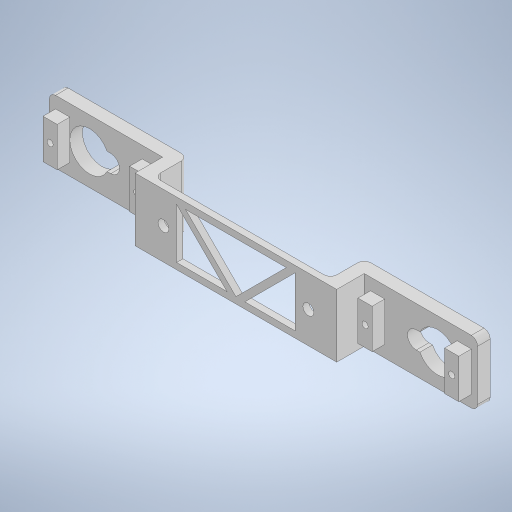
# Autodesk Inventor part: axis2
Saved by Autodesk Inventor 2023 (Build 270158000, 158)
## iProperties
Created: 2023-04-29
Part Number: axis2
Material: 一般
Document SubType Name: Modeling
Designer: taka2
Density: 1 g/cm^3
Appearance: 既定
Author: taka2
Autodesk Inventor part; units mm, degrees
ref_plane "YZ Plane" through (0, 0, 0) normal (1, 0, 0) x (0, 1, 0)
ref_plane "XZ Plane" through (0, 0, 0) normal (0, 1, 0) x (-1, 0, 0)
ref_plane "XY Plane" through (0, 0, 0) normal (0, 0, 1) x (1, 0, 0)
sketch "スケッチ1" plane through (0, 0, 0) normal (0, 0, 1) x (1, 0, 0)
  line L0 (-12.75, -10) -> (27.25, -10)
  line L1 (27.25, -10) -> (27.25, 10)
  line L2 (27.25, 10) -> (-12.75, 10)
  line L3 (-12.75, 10) -> (-12.75, -10)
  line L4 (-10.75, 6.25) -> (21.25, 6.25)
  line L5 (21.25, 6.25) -> (21.25, -6.25)
  line L6 (21.25, -6.25) -> (-10.75, -6.25)
  line L7 (-10.75, -6.25) -> (-10.75, 6.25)
  line L8 (0, 14.1006) -> (0, -12.8692)
  line L9 (-16.3835, 0) -> (166.3597, 0)
  line L10 (-6.25, 6.25) -> (-6.25, -6.25)
  line L11 (16.75, 6.25) -> (16.75, -6.25)
  arc A0 (5.5877, 2.8) -> (5.5877, -2.8) centre (0, 0) ccw
  arc A1 (6.75, -2.8) -> (6.75, 2.8) centre (6.75, 0) ccw
  line L12 (6.75, 2.8) -> (5.5877, 2.8)
  line L13 (6.75, -2.8) -> (5.5877, -2.8)
  circle A2 centre (-8.5, 0) radius 1
  circle A3 centre (19, 0) radius 1
  line L14 (23.25, 10) -> (23.25, -10)
  point P0 (-6.25, 0)
  dimension "d0" = 4.5
  dimension "d1" = 4.5
  dimension "d2" = 12.5
  dimension "d3" = 2.8
  dimension "d4" = 13
  dimension "d5" = 23
  dimension "d6" = 2
  dimension "d7" = 2.25
  dimension "d8" = 2.25
  dimension "d9" = 20
  dimension "d10" = 2
  dimension "d29" = 2
  dimension "d30" = 4
  constraints: 30 end point, 11 point on line, 6 parallel, 5 perpendicular, 4 centre point, 4 point on circle, 4 tangent, 3 horizontal, 1 coincident, 1 equal radius, 1 vertical, 2 other
  measures "d0" distance of L6.end L10.end
  measures "d1" distance of L5.end L11.end
  measures "d2" distance of L4.end L5.end
  measures "d3" radius of A1
  measures "d4" distance from line of A1.centre L10
  measures "d5" distance of L11.end L10.end
  measures "d6" diameter of A3
  measures "d7" distance from line of L5 A3.centre
  measures "d8" distance from line of L7 A2.centre
  measures "d9" distance of L2.end L0.start
  measures "d10" distance between parallel lines of L3 L7
  measures "d29" distance between parallel lines of L14 L5
  measures "d30" distance between parallel lines of L1 L14
extrude "押し出し1" add sketch "スケッチ1" along normal blind 4 contours L14 L9 L1 L0 | L0 L8 L6 L5 L9 L14 | L0 L3 L9 L7 L6 L8 | L14 L2 L1 L9 | L9 L5 L4 L8 L2 L14 | A0 L13 A1 L9 L11 L6 | L6 L10 A0 | L3 L2 L8 L4 L7 L9 | L10 L4 A0 | L9 A1 L12 A0 L4 L11
extrude "押し出し2" add sketch "スケッチ1" along normal blind 8 contours L9 A3 L11 L4 L5 | L5 L6 L11 L9 A3 | L6 L7 L9 A2 L10 | L9 A2 L7 L4 L10
extrude "押し出し4" add sketch "スケッチ1" along normal blind 12.75 contours L14 L9 L1 L0 | L14 L2 L1 L9
sketch "スケッチ2" plane through (0, 0, 12.75) normal (0, 0, 1) x (1, 0, 0)
  line L0 (23.25, -10) -> (23.25, 10) projected
  line L1 (23.25, 0) -> (87.25, 0)
  line L2 (23.25, 10) -> (87.25, 10)
  line L3 (87.25, 10) -> (87.25, -10)
  line L4 (87.25, -10) -> (23.25, -10)
  line L5 (36.4216, 8) -> (36.4216, -8)
  line L6 (36.4216, -8) -> (52.4216, -8)
  line L7 (52.4216, -8) -> (36.4216, 8)
  line L8 (39.25, 8) -> (55.25, -8)
  line L9 (55.25, -8) -> (71.25, 8)
  line L10 (71.25, 8) -> (39.25, 8)
  line L11 (58.0784, -8) -> (74.0784, 8)
  circle A0 centre (32.25, 0) radius 1.75
  circle A1 centre (32.25, 0) radius 3
  line L12 (27.25, -10) -> (27.25, 10) projected
  line L13 (83.25, 10) -> (83.25, -10)
  line L14 (74.0784, 8) -> (74.0784, -8)
  line L15 (58.0784, -8) -> (74.0784, -8)
  line L16 (55.25, 10) -> (55.25, -10)
  circle A2 centre (78.25, 0) radius 1.75
  circle A3 centre (78.25, 0) radius 3
  point P0 (0, 0)
  dimension "d33" = 3.5
  dimension "d34" = 6
  dimension "d37" = 16
  dimension "d38" = 2
  dimension "d39" = 2
  dimension "d43" = 4
  dimension "d63" = 64
  dimension "d64" = 46
  constraints: 30 end point, 7 point on line, 5 equal length, 4 centre point, 4 horizontal, 4 midpoint, 4 perpendicular, 3 symmetric about line, 2 coincident, 2 vertical, 1 parallel, 2 other
  measures "d33" diameter of A0
  measures "d34" diameter of A1
  measures "d37" distance of L5.start L5.end
  measures "d38" distance between parallel lines of L8 L7
  measures "d39" distance between parallel lines of L11 L9
  measures "d43" distance between parallel lines of L3 L13
  measures "d63" distance between parallel lines of L3 L0
  measures "d64" distance of A2.centre A0.centre
extrude "押し出し5" add sketch "スケッチ2" against normal blind 2 contours L12 L1 A1 L5 L6 L7 L8 L16 L4 | L12 L2 L16 L10 L8 L1 L7 L5 A1 | L16 L9 L1 L11 L15 L14 A3 L13 L4 | A1 L1 A0 | L1 A0 A1 | L2 L13 L1 A3 L14 L11 L9 L10 L16 | A3 L1 A2 | L1 A2 A3
extrude "押し出し6" add sketch "スケッチ2" against normal blind 12.75 contours L13 L1 L3 L4 | L13 L2 L3 L1
sketch "スケッチ3" plane through (0, 0, 0) normal (0, 0, 1) x (1, 0, 0)
  line L0 (83.25, 10) -> (83.25, -10) projected
  line L1 (83.25, 10) -> (123.25, 10)
  line L2 (123.25, 10) -> (123.25, -10)
  line L3 (123.25, -10) -> (83.25, -10)
  line L4 (121.25, 6.25) -> (89.25, 6.25)
  line L5 (89.25, 6.25) -> (89.25, -6.25)
  line L6 (89.25, -6.25) -> (121.25, -6.25)
  line L7 (121.25, -6.25) -> (121.25, 6.25)
  line L8 (93.75, 6.25) -> (93.75, -6.25)
  line L9 (116.75, 6.25) -> (116.75, -6.25)
  line L10 (87.25, -10) -> (87.25, 10) projected
  line L11 (87.25, 0) -> (123.25, 0)
  arc A0 (104.9123, -2.8) -> (104.9123, 2.8) centre (110.5, 0) ccw
  arc A1 (103.75, 2.8) -> (103.75, -2.8) centre (103.75, 0) ccw
  line L12 (103.75, 2.8) -> (104.9123, 2.8)
  line L13 (103.75, -2.8) -> (104.9123, -2.8)
  circle A2 centre (119, 0) radius 1
  circle A3 centre (91.5, 0) radius 1
  point P0 (0, 0)
  point P1 (116.75, 0)
  dimension "d48" = 2
  dimension "d49" = 12.5
  dimension "d50" = 4.5
  dimension "d51" = 4.5
  dimension "d52" = 2.25
  dimension "d53" = 2.25
  dimension "d54" = 23
  dimension "d55" = 13
  dimension "d56" = 2.8
  dimension "d57" = 2
  dimension "d58" = 2
  constraints: 24 end point, 8 point on line, 4 centre point, 4 horizontal, 4 perpendicular, 4 point on circle, 3 tangent, 2 midpoint, 2 parallel, 1 equal radius, 2 other
  measures "d48" diameter of A2
  measures "d49" distance of L6.end L4.start
  measures "d50" distance of L9.end L6.end
  measures "d51" distance of L8.end L5.end
  measures "d52" distance from line of L7 A2.centre
  measures "d53" distance from line of L5 A3.centre
  measures "d54" distance of L9.end L8.end
  measures "d55" distance from line of A1.centre L9
  measures "d56" radius of A1
  measures "d57" distance between parallel lines of L5 L10
  measures "d58" distance between parallel lines of L2 L7
extrude "押し出し7" add sketch "スケッチ3" along normal blind 4 contours L1 L2 L11 L7 L4 L5 L10 | L10 L11 L5 L6 L7 L2 L3 | L4 A0 L12 A1 L11 L8 | L8 L11 A1 L13 A0 L6 | L6 A0 L9 | L9 A0 L4
extrude "押し出し8" add sketch "スケッチ3" along normal blind 8 contours L11 A3 L8 L6 L5 | L5 L4 L8 L11 A3 | L11 A2 L9 L4 L7 | L7 L6 L9 L11 A2
fillet "フィレット1" radius 2 4 edges at (-12.75, 10, 2) (-12.75, -10, 2) (123.25, -10, 2) (123.25, 10, 2)
fillet "フィレット2" radius 2 4 edges at (27.25, 0, 0) (27.25, 0, 10.75) (83.25, 0, 0) (83.25, 0, 10.75)
